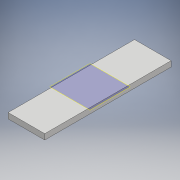
# Autodesk Inventor part: base oreja
Saved by Autodesk Inventor 2017 (Build 210142000, 142)
## iProperties
Part Number: base oreja
Material: Genérico
Document SubType Name: Chapa
Designer: Kevin
Density: 1 g/cm^3
Sheet Metal Rule: Por defecto_mm
Appearance: Valor por defecto
Author: Kevin
Autodesk Inventor part; units mm, degrees
ref_plane "YZ Plane" through (0, 0, 0) normal (1, 0, 0) x (0, 1, 0)
ref_plane "XZ Plane" through (0, 0, 0) normal (0, 1, 0) x (-1, 0, 0)
ref_plane "XY Plane" through (0, 0, 0) normal (0, 0, 1) x (1, 0, 0)
ref_plane "Plano de trabajo1" through (0, 0, 0) normal (0, 0, -1) x (-1, 0, 0)
sketch "Boceto6" plane through (0, 0, 0) normal (0, 0, -1) x (-1, 0, 0)
  line L0 (10.2083, 22.272) -> (10.2083, 34.5)
  line L1 (-9.7917, -34.5) -> (-9.7917, 34.5)
  line L2 (10.2083, -34.5) -> (10.2083, 22.272)
  line L3 (-0.0082, 34.5) -> (10.2083, 34.5)
  line L4 (-0.0082, 34.5) -> (-9.7917, 34.5)
  line L5 (-0.037, -34.5) -> (10.2083, -34.5)
  line L6 (-0.037, -34.5) -> (-9.7917, -34.5)
  constraints: 14 end point, 3 perpendicular, 2 vertical, 1 point on line
extrude "Extrusión4" add sketch "Boceto6" along normal blind 3
equation "\"Radio_pliegue\" = Grosor"
equation "\"Anchura_desahogo_plegado\" = Grosor"
equation "\"Profundidad_desahogo_plegado\" = 0.5 * Grosor"
equation "\"Tamaño_destalonado\" = 4 * Grosor"
equation "\"Remanente_mínimo\" = 2 * Grosor"
equation "\"Radiodetransición\" = Radio_pliegue"
equation "\"Tamaño_de_radio_de_Jacobi\" = Radio_pliegue"
equation "\"TamañoSeparación\" = Grosor"
equation "\"Grosor\" = 0.5"
